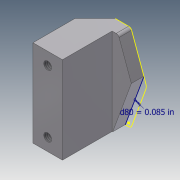
# Autodesk Inventor part: J005413
Saved by Autodesk Inventor 2018.2 (Build 222227000, 227)
## iProperties
Created: 2015-10-29
Material: ALUMINUM, 6061-T651
Vendor: HHMI: JRC - ID&F
Document SubType Name: Modeling
Designer: ARNOLDJ
Density: 2.7 g/cm^3
Appearance: Metal-AL-6061 (Machined)
Mass: 30.2831 g
Surface Area: 38.979 cm^2
Volume: 11.216 cm^3
Part Number: J005413
Description: HARD STOP FOR POSITIONER ROTARY STAGE
Project: P-201804
RuleStatus: InUse
AfterDocSave0: file://Part Number Cleaner
LAB/DEPT: SVOBODA (LAB)
REQUESTING SCIENTIST: SOFRONIEW, NICK
SURFACE ROUGHNESS: 63 Ra
DESIGN DEPARTMENT: HHMI: JRC - ID&F
SPECIAL FINISH: ANODIZE PER MIL-A-8625F, TYPE II, CLASS 2 (BLACK)
ALTERED ITEM PART NUMBER: N/A
ALTERED ITEM VENDOR: N/A
ALTERED ITEM DESCRIPTION: N/A
Author: ARNOLDJ
Revision Number: A
Autodesk Inventor part; units mm, degrees
ref_plane "YZ Plane" through (0, 0, 0) normal (1, 0, 0) x (0, 1, 0)
ref_plane "XZ Plane" through (0, 0, 0) normal (0, 1, 0) x (-1, 0, 0)
ref_plane "XY Plane" through (0, 0, 0) normal (0, 0, 1) x (1, 0, 0)
sketch "Sketch1" plane through (0, 0, 0) normal (0, 0, 1) x (1, 0, 0)
  line L0 (6.0325, -17.78) -> (-6.0325, -17.78)
  line L1 (-6.0325, -17.78) -> (-6.0325, 17.78)
  line L2 (-6.0325, 17.78) -> (6.0325, 17.78)
  line L3 (6.0325, 17.78) -> (6.0325, -17.78)
  line L4 (6.0325, -17.78) -> (-6.0325, 17.78) construction
  line L5 (-6.0325, -17.78) -> (6.0325, 17.78) construction
  point P0 (0, 0)
  dimension "d0" = 12.065
  dimension "d1" = 35.56
  constraints: 12 end point, 2 midpoint, 2 parallel, 1 horizontal, 1 perpendicular
  measures "d0" distance of L1.end L2.end
  measures "d1" distance of L0.end L1.end
extrude "Extrusion1" add sketch "Sketch1" along normal blind 25.4
sketch "Sketch3" plane through (0, 0, 25.4) normal (0, 0, 1) x (1, 0, 0)
  line L0 (6.0325, -17.78) -> (6.0325, 17.78) projected
  line L1 (0, 26.67) -> (0, -26.67) projected
  line L2 (-8.4455, 0) -> (8.4455, 0) projected
  point P0 (0, 12.7)
  point P1 (0, -12.7)
  dimension "d45" = 12.7
  dimension "d46" = 12.7
  dimension "d47" = 0
  constraints: 1 vertical alignment
  measures "d45" distance from line of L2 point (0, 12.7)
  measures "d46" distance from line of L2 point (0, -12.7)
  measures "d47" distance from line of L1 point (0, 12.7)
hole "Hole5" at (0, 12.7, 25.4) at (0, -12.7, 25.4) direction (0, 0, -1) diameter 3.2512 depth 11.811 tip angle 118
sketch "Sketch7" plane through (0, 0, 0) normal (0, 0, -1) x (-1, 0, 0)
  line L0 (-6.0325, -17.78) -> (6.0325, -17.78) projected
  line L1 (6.0325, 17.78) -> (-6.0325, 17.78) projected
  line L2 (-6.0325, 17.78) -> (-6.0325, -17.78) projected
  line L3 (-15.0439, 0) -> (-8.5725, -17.78)
  line L4 (-6.0325, -17.78) -> (-8.5725, -17.78)
  line L5 (-15.0439, 0) -> (-8.5725, 17.78)
  line L6 (-8.5725, 17.78) -> (-6.0325, 17.78)
  line L7 (0, -26.67) -> (0, 26.67) projected
  line L8 (-19.0666, 0) -> (10.2157, 0) projected
  point P0 (0, 0)
  dimension "d70" = 70
  dimension "d71" = 70
  dimension "d72" = 2.54
  constraints: 8 end point, 2 horizontal, 1 point on line
  measures "d70" angle of L8 L3
  measures "d71" angle of L8 L5
  measures "d72" distance of L0.start L3.end
extrude "Extrusion6" add sketch "Sketch7" against normal blind 5.08 contours L4 L3 L8 L2 | L8 L5 L6 L2
fillet "Fillet1" radius 3.175 1 edges at (15.0439, 0, 2.54)
fillet "Fillet2" radius 1.27 2 edges at (8.5725, -17.78, 2.54) (8.5725, 17.78, 2.54)
chamfer "Chamfer1" distance 8.255 angle 45 1 edges at (-6.0325, 0, 0)
sketch "Sketch8" plane through (0, 0, 0) normal (0, 0, -1) x (-1, 0, 0)
  line L0 (-2.2225, 17.78) -> (-2.2225, -17.78) projected
  line L1 (-2.2225, 17.78) -> (-7.6832, 17.78) projected
  arc A0 (-7.6832, 17.78) -> (-8.8766, 16.9444) centre (-7.6832, 16.51) ccw projected
  line L2 (-8.8766, 16.9444) -> (-14.6487, 1.0859) projected
  arc A1 (-14.6487, 1.0859) -> (-14.6487, -1.0859) centre (-11.6651, 0) ccw projected
  line L3 (-14.6487, -1.0859) -> (-8.8766, -16.9444) projected
  arc A2 (-8.8766, -16.9444) -> (-7.6832, -17.78) centre (-7.6832, -16.51) ccw projected
  line L4 (-7.6832, -17.78) -> (-2.2225, -17.78) projected
  line L5 (-14.6487, 1.0859) -> (-8.8766, 16.9444) projected
  line L6 (-13.8951, 3.1562) -> (-6.2749, -17.78)
  line L7 (-14.6487, -1.0859) -> (-8.8766, -16.9444) projected
  point P0 (0, 0)
  dimension "d80" = 2.159
  constraints: 2 end point, 2 point on line, 1 parallel
  measures "d80" distance between parallel lines of L6 L3
extrude "Extrusion7" cut sketch "Sketch8" against normal up to next contours L4 A2 L3 A1 L2 L6
body "Solid1"
